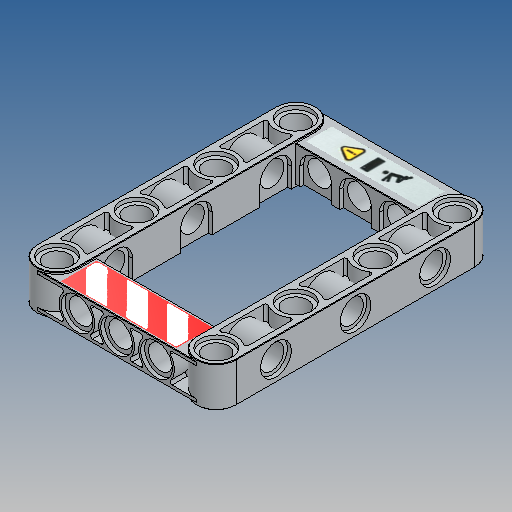
# Autodesk Inventor part: 64179-LtBluishGray
Saved by Autodesk Inventor 2025 (Build 290162010, 162A)
## iProperties
Created: 2012-03-21
Part Number: 64179-LtBluishGray
Document SubType Name: Modeling
Designer: D. Kohfeld
Density: 1.06 g/cm^3
Material: ABS Plastic
Mass: 5.69641 g
Surface Area: 80.0064 cm^2
Volume: 5.37397 cm^3
Appearance: LtBluishGray
Author: D. Kohfeld
Autodesk Inventor part; units mm, degrees
ref_plane "XZ Plane" through (0, 0, 0) normal (0, 1, 0) x (-1, 0, 0)
ref_plane "XY Plane" through (0, 0, 0) normal (0, 0, 1) x (1, 0, 0)
sketch "Sketch1" plane through (0, 0, 0) normal (0, 0, 1) x (1, 0, 0)
  line L0 (4, -24) -> (4, 24)
  line L1 (-4, 24) -> (-4, -24)
  arc A0 (4, 24) -> (-4, 24) centre (0, 24) ccw
  arc A1 (-4, -24) -> (4, -24) centre (0, -24) ccw
  circle A2 centre (0, 24) radius 3.2
  circle A3 centre (0, 24) radius 2.4
  line L2 (2.8284, 21.1716) -> (2.8284, 10.8284)
  line L3 (-2.8284, 21.1716) -> (-2.8284, 10.8284)
  arc A4 (-2.8284, 21.1716) -> (2.8284, 21.1716) centre (0, 24) ccw
  arc A5 (2.8284, 10.8284) -> (-2.8284, 10.8284) centre (0, 8) ccw
  circle A6 centre (0, 8) radius 3.2
  circle A7 centre (0, 8) radius 2.4
  line L4 (2.8284, 5.1716) -> (2.8284, -5.1716)
  line L5 (-2.8284, 5.1716) -> (-2.8284, -5.1716)
  arc A8 (-2.8284, 5.1716) -> (2.8284, 5.1716) centre (0, 8) ccw
  arc A9 (2.8284, -5.1716) -> (-2.8284, -5.1716) centre (0, -8) ccw
  circle A10 centre (0, -8) radius 3.2
  circle A11 centre (0, -8) radius 2.4
  line L6 (2.8284, -10.8284) -> (2.8284, -21.1716)
  line L7 (-2.8284, -10.8284) -> (-2.8284, -21.1716)
  arc A12 (-2.8284, -10.8284) -> (2.8284, -10.8284) centre (0, -8) ccw
  arc A13 (2.8284, -21.1716) -> (-2.8284, -21.1716) centre (0, -24) ccw
  circle A14 centre (0, -24) radius 3.2
  circle A15 centre (0, -24) radius 2.4
  line L8 (0, 24) -> (-2.8284, 21.1716) construction
  point P0 (0, 0)
  point P1 (-4, 0)
  dimension "d48" = 48
  dimension "d49" = 6.4
  dimension "d50" = 4.8
  dimension "d51" = 16
  dimension "d64" = 16
  dimension "d116" = 45
  dimension "d117" = 56
  dimension "d118" = 8
  constraints: 18 end point, 16 centre point, 16 point on circle, 9 coincident, 4 equal radius, 4 tangent, 3 horizontal alignment, 3 vertical, 2 vertical alignment, 1 midpoint, 1 parallel, 28 other
  measures "d48" distance of A1.centre A0.centre
  measures "d49" diameter of A2
  measures "d50" diameter of A3
  measures "d51" distance of A0.centre A5.centre
  measures "d64" distance of L3.start L5.start
  measures "d116" angle of L8 L1
  measures "d118" diameter of A0
extrude "Extrusion1" add sketch "Sketch1" along normal mid plane 8 contours A1 L1 A0 L0 | A2 | L2 A5 L3 A4 | A6 | L4 A9 L5 A8 | A10 | L6 A13 L7 A12 | A14
sketch "Sketch6" plane through (0, 0, 4) normal (0, 0, 1) x (1, 0, 0)
  circle A0 centre (0, 24) radius 2.4 projected
  circle A1 centre (0, 24) radius 3.2 projected
  line L0 (2.8284, 21.1716) -> (2.8284, 10.8284) projected
  arc A2 (-2.8284, 21.1716) -> (2.8284, 21.1716) centre (0, 24) ccw projected
  arc A3 (2.8284, 10.8284) -> (-2.8284, 10.8284) centre (0, 8) ccw projected
  line L1 (-2.8284, 21.1716) -> (-2.8284, 10.8284) projected
  circle A4 centre (0, 8) radius 3.2 projected
  circle A5 centre (0, 24) radius 3.1 projected
  circle A6 centre (0, 8) radius 3.1 projected
  line L2 (4, 24) -> (4, -24) projected
  line L3 (4, -24) -> (4, 24) projected
  arc A7 (-2.8284, 5.1716) -> (2.8284, 5.1716) centre (0, 8) ccw projected
  line L4 (2.8284, 5.1716) -> (2.8284, -5.1716) projected
  arc A8 (2.8284, -5.1716) -> (-2.8284, -5.1716) centre (0, -8) ccw projected
  line L5 (-2.8284, 5.1716) -> (-2.8284, -5.1716) projected
  circle A9 centre (0, -8) radius 3.2 projected
  line L6 (2.8284, -10.8284) -> (2.8284, -21.1716) projected
  arc A10 (-2.8284, -10.8284) -> (2.8284, -10.8284) centre (0, -8) ccw projected
  line L7 (-2.8284, -10.8284) -> (-2.8284, -21.1716) projected
  arc A11 (2.8284, -21.1716) -> (-2.8284, -21.1716) centre (0, -24) ccw projected
  circle A12 centre (0, -24) radius 3.2 projected
extrude "Extrusion7" cut sketch "Sketch6" against normal blind 0.8 contours A0 | A1 | A4 | A5 | A6 | A9 | A12
extrude "Extrusion8" cut sketch "Sketch6" against normal blind 3.1 contours L0 A3 L1 A2 | A7 L4 A8 L5 | L6 A11 L7 A10
sketch "Sketch15" plane through (0, 0, -4) normal (0, 0, -1) x (-1, 0, 0)
  circle A0 centre (0, -8) radius 2.4 projected
  circle A1 centre (0, 8) radius 2.4 projected
  arc A2 (4, 24) -> (-4, 24) centre (0, 24) ccw projected
  line L0 (-4, -24) -> (-4, 24) projected
  arc A3 (-4, -24) -> (4, -24) centre (0, -24) ccw projected
  line L1 (4, 24) -> (4, -24) projected
  line L2 (-2.8284, -5.1716) -> (-2.8284, 5.1716)
  arc A4 (2.4, -4.8) -> (-2.8284, -5.1716) centre (0, -8) ccw
  arc A5 (-2.8284, 5.1716) -> (2.4, 4.8) centre (0, 8) ccw
  line L3 (2.4, 4.8) -> (2.4, -4.8)
  line L4 (0, -8) -> (-2.8284, -5.1716) construction
  line L5 (-2.8284, -21.1716) -> (-2.8284, -10.8284)
  line L6 (2.4, -20.8) -> (2.4, -11.2)
  arc A6 (2.4, -20.8) -> (-2.8284, -21.1716) centre (0, -24) ccw
  arc A7 (-2.8284, -10.8284) -> (2.4, -11.2) centre (0, -8) ccw
  line L7 (-2.8284, 10.8284) -> (-2.8284, 21.1716)
  line L8 (2.4, 11.2) -> (2.4, 20.8)
  arc A8 (2.4, 11.2) -> (-2.8284, 10.8284) centre (0, 8) ccw
  arc A9 (-2.8284, 21.1716) -> (2.4, 20.8) centre (0, 24) ccw
  point P0 (0, 0)
  dimension "d109" = 45
  dimension "d111" = 1.6
  constraints: 14 end point, 12 point on circle, 6 centre point, 6 coincident, 6 equal radius, 6 parallel, 4 vertical alignment, 1 vertical
  measures "d109" angle of L0 L4
  measures "d111" distance between parallel lines of L1 L6
extrude "Extrusion19" cut sketch "Sketch15" against normal blind 3.1 contours L2 A5 L3 A4 | L5 A7 L6 A6 | L7 A9 L8 A8
mirror "Mirror5" about plane through (0, 0, 0) normal (0, 0, 1) of "Extrusion7"
sketch "Sketch7" plane through (0, 0, 0) normal (1, 0, 0) x (0, 1, 0)
  circle A0 centre (-16, 0) radius 3.6
  circle A1 centre (-16, 0) radius 2.4
  circle A2 centre (0, 0) radius 3.6
  circle A3 centre (0, 0) radius 2.4
  circle A4 centre (16, 0) radius 3.6
  circle A5 centre (16, 0) radius 2.4
  line L0 (-16, 0) -> (0, 0) construction
  line L1 (0, 0) -> (16, 0) construction
  dimension "d69" = 7.2
  dimension "d70" = 4.8
  dimension "d114" = 16
  constraints: 6 centre point, 4 coincident, 4 end point, 4 equal radius, 2 collinear, 1 horizontal alignment
  measures "d69" diameter of A0
  measures "d70" diameter of A1
  measures "d114" distance of L0.start L0.end
extrude "Extrusion9" add sketch "Sketch7" against normal up to surface (8 mm away) from surface at 4
extrude "Extrusion10" cut sketch "Sketch7" along normal through all both and the other way through all contours A1 | A3 | A5
sketch "Sketch8" plane through (4, -24, 4) normal (1, 0, 0) x (0, 0, -1)
  circle A0 centre (4, 24) radius 2.4 projected
  circle A1 centre (4, 8) radius 2.4 projected
  circle A2 centre (4, 40) radius 2.4 projected
  circle A3 centre (4, 8) radius 3.1
  circle A4 centre (4, 24) radius 3.1
  circle A5 centre (4, 40) radius 3.1
  dimension "d75" = 6.2
  constraints: 3 centre point, 3 coincident, 2 equal radius
  measures "d75" diameter of A3
extrude "Extrusion11" cut sketch "Sketch8" against normal blind 0.8
sketch "Sketch14" plane through (-4, -24, 4) normal (-1, 0, 0) x (0, 0, 1)
  circle A0 centre (-4, 24) radius 2.4 projected
  circle A1 centre (-4, 8) radius 2.4 projected
  circle A2 centre (-4, 40) radius 2.4 projected
  line L0 (-8, 48) -> (-8, 0) projected
  line L1 (-8, 0) -> (0, 0) projected
  line L2 (-8, 43.2) -> (-4, 43.2)
  arc A3 (-4, 36.8) -> (-4, 43.2) centre (-4, 40) ccw
  line L3 (-4, 36.8) -> (-8, 36.8)
  line L4 (-8, 27.2) -> (-4, 27.2)
  arc A4 (-4, 20.8) -> (-4, 27.2) centre (-4, 24) ccw
  line L5 (-4, 20.8) -> (-8, 20.8)
  line L6 (-8, 11.2) -> (-4, 11.2)
  arc A5 (-4, 4.8) -> (-4, 11.2) centre (-4, 8) ccw
  line L7 (-4, 4.8) -> (-8, 4.8)
  dimension "d106" = 6.4
  constraints: 12 end point, 6 point on circle, 6 point on line, 6 tangent, 3 centre point, 3 concentric, 3 parallel, 3 perpendicular, 2 equal radius
  measures "d106" diameter of A3
extrude "Extrusion18" cut sketch "Sketch14" against normal blind 0.8
fillet "Fillet2" radius 0.4 24 edges at (-2.8284, 21.1716, 2.45) (-2.8284, 10.8284, 2.45) (2.8284, 10.8284, 2.45) (2.8284, 21.1716, 2.45) (-2.8284, -21.1716, 2.45) (-2.8284, -10.8284, 2.45) (2.8284, -10.8284, 2.45) (2.8284, -21.1716, 2.45) (2.8284, -5.1716, 2.45) (-2.8284, -5.1716, 2.45) (-2.8284, 5.1716, 2.45) (2.8284, 5.1716, 2.45) (-2.4, 20.8, -2.45) (2.8284, 21.1716, -2.45) (2.8284, 10.8284, -2.45) (-2.4, 11.2, -2.45) (-2.4, 4.8, -2.45) (2.8284, 5.1716, -2.45) (-2.4, -4.8, -2.45) (2.8284, -5.1716, -2.45) (-2.4, -11.2, -2.45) (2.8284, -10.8284, -2.45) (2.8284, -21.1716, -2.45) (-2.4, -20.8, -2.45)
fillet "Fillet2" radius 0.1 11 edges at (-4, 0, 4) (0, 28, 4) (4, 0, 4) (0, -28, 4) (0, 28, -4) (-4, 8, -4) (-4, -8, -4) (-4, -21.6, -4) (-4, 21.6, -4) (0, -28, -4) (4, 0, -4)
ref_plane "Work Plane1" through (-16, 0, 0) normal (1, 0, 0) x (0, 1, 0)
sketch "Sketch11" plane through (-16, 0, 0) normal (1, 0, 0) x (0, 1, 0)
  line L0 (-28, -3.9) -> (-28, 3.9) construction
  line L1 (-28, -3.6) -> (-20, -3.6)
  line L2 (-20, -3.6) -> (-20, 3.6)
  line L3 (-20, 3.6) -> (-28, 3.6)
  line L4 (-28, 3.6) -> (-28, 2.9)
  line L5 (-28, 2.9) -> (-24.9, 2.9)
  line L6 (-24.9, 2.9) -> (-24.9, -2.9)
  line L7 (-24.9, -2.9) -> (-28, -2.9)
  line L8 (-28, -2.9) -> (-28, -3.6)
  point P0 (0, 0)
  point P1 (-20, 0)
  point P2 (-28, 0)
  dimension "d86" = 8
  dimension "d87" = 3.1
  dimension "d88" = 5.8
  dimension "d89" = 7.2
  constraints: 16 end point, 6 perpendicular, 4 point on line, 2 collinear, 2 midpoint, 1 horizontal alignment
  measures "d86" distance between parallel lines of L2 L0
  measures "d87" distance between parallel lines of L0 L6
  measures "d88" distance between parallel lines of L7 L5
  measures "d89" distance between parallel lines of L1 L3
extrude "Extrusion13" add sketch "Sketch11" along normal up to next
sketch "Sketch12" plane through (-16, -28, 2.9) normal (0, -1, 0) x (1, 0, 0)
  line L0 (0, 0.7) -> (16, 0.7) projected
  line L1 (0, 0.7) -> (0, 0) projected
  line L2 (16, -6.5) -> (16, -5.8) projected
  line L3 (0, -5.8) -> (16, -5.8) projected
  line L4 (0, -5.8) -> (0, -6.5) projected
  line L5 (0, -6.5) -> (16, -6.5) projected
  circle A0 centre (8, -2.9) radius 3.6
  circle A1 centre (8, -2.9) radius 2.4
  circle A2 centre (8, -2.9) radius 3.2
  arc A3 (0, -6.5) -> (0, 0.7) centre (0, -2.9) ccw
  arc A4 (0, -6.1) -> (0, 0.3) centre (0, -2.9) ccw
  circle A5 centre (0, -2.9) radius 2.4
  line L6 (0, -2.9) -> (8, -2.9) construction
  line L7 (8, -2.9) -> (16, -2.9) construction
  line L8 (0, -6.5) -> (0, 0.7)
  dimension "d92" = 4.8
  dimension "d93" = 6.4
  constraints: 6 centre point, 6 end point, 4 coincident, 4 point on circle, 4 tangent, 3 collinear, 2 equal radius, 2 point on line, 1 horizontal alignment, 1 parallel
  measures "d92" diameter of A5
  measures "d93" diameter of A4
extrude "Extrusion14" add sketch "Sketch12" against normal up to surface (3.1 mm away) contours A3 L3 A4 L1 | A0 L3 A2 | A4 L3 L8 A5 L1 | A3 L4 A4 L3 | L3 A2 A0 | A4 L4 L3 | A2 L3 | L3 A2 | A5 L8 picked at (0.4988, -2.2745)
extrude "Extrusion15" cut sketch "Sketch12" against normal through all contours L8 A5 | A5 L8 | A1
extrude "Extrusion16" cut sketch "Sketch12" against normal blind 0.8 contours A4 L3 L8 A5 L1 | A4 L4 L3 | A2 L3 | L3 A2 | A5 L8 picked at (0.4988, -2.2745)
sketch "Sketch13" plane through (-16, -20, 3.6) normal (0, 1, 0) x (1, 0, 0)
  arc A0 (0, 1.2) -> (0, 6) centre (0, 3.6) ccw projected
  line L0 (0, 1.2) -> (0, 0) projected
  line L1 (0, 7.2) -> (12, 7.2) projected
  line L2 (0, 7.2) -> (0, 6) projected
  circle A1 centre (8, 3.6) radius 2.4 projected
  line L3 (3.2, 7.2) -> (3.2, 3.6)
  arc A2 (0, 0.4) -> (3.2, 3.6) centre (0, 3.6) ccw
  arc A3 (4.8, 3.6) -> (11.2, 3.6) centre (8, 3.6) ccw
  line L4 (4.8, 3.6) -> (4.8, 7.2)
  line L5 (11.2, 3.6) -> (11.2, 7.2)
  point P0 (16, 3.6)
  dimension "d100" = 6.4
  constraints: 6 end point, 4 point on circle, 4 point on line, 3 tangent, 2 centre point, 2 coincident, 2 perpendicular, 1 equal radius, 1 parallel
  measures "d100" diameter of A3
extrude "Extrusion17" cut sketch "Sketch13" against normal blind 0.8
fillet "Fillet3" radius 0.1 7 edges at (-4, -28, 3.6) (-12, -28, 3.6) (-10, -20, 3.6) (-12, -28, -3.6) (-4, -28, -3.6) (-4.4, -20, -3.6) (-12, -20, -3.6)
fillet "Fillet3" radius 0.4 6 edges at (-5.8669, -26.45, -2.9) (-5.8669, -26.45, 2.9) (-10.1331, -26.45, 2.9) (-10.1331, -26.45, -2.9) (-13.8669, -26.45, -2.9) (-13.8669, -26.45, 2.9)
mirror "Mirror4" about plane through (0, 0, 0) normal (0, 1, 0) of "Extrusion13", "Extrusion14", "Extrusion16", "Extrusion17", "Extrusion15", "Fillet3"
mirror "Mirror3" about plane through (-16, 0, 0) normal (1, 0, 0) of "Extrusion7", "Extrusion1", "Extrusion11", "Extrusion10", "Extrusion9", "Extrusion8", "Fillet2", "Extrusion13", "Extrusion14", "Extrusion16", "Extrusion17", "Extrusion15", "Mirror4", "Fillet3", "Extrusion19", "Extrusion18", "Mirror5"
sketch "Skizze16" plane through (-4, -24, 3.6) normal (0, 0, 1) x (1, 0, 0)
  line L0 (-23.3393, 50.6) -> (-0.6607, 50.6) construction
  line L1 (-0.6607, 50.6) -> (-0.6607, 45.4) construction
  line L2 (-0.6607, 45.4) -> (-23.3393, 45.4) construction
  line L3 (-23.3393, 45.4) -> (-23.3393, 50.6) construction
  line L4 (-28, -4) -> (4, -4) projected
  line L5 (4, 52) -> (-28, 52) projected
  line L6 (-24, 44) -> (0, 44) projected
  line L7 (-27.1112, 51.9) -> (3.1112, 51.9) projected
  point P0 (4, 24)
  point P1 (-12, 50.6)
  point P2 (-14.8102, 48.9)
  point P3 (-12, 51.9)
  dimension "d146" = 1.4
  dimension "d147" = 1.4
  constraints: 2 midpoint, 1 vertical alignment, 2 other
  measures "d146" distance between parallel lines of L5 L0
  measures "d147" distance between parallel lines of L2 L6
decal "Aufkleber1"
sketch "Skizze17" plane through (-4, 20.1, 3.6) normal (0, 0, 1) x (1, 0, 0)
  line L0 (-23.6033, -40.5) -> (-0.3967, -40.5) construction
  line L1 (-0.3967, -40.5) -> (-0.3967, -47.7) construction
  line L2 (-0.3967, -47.7) -> (-23.6033, -47.7) construction
  line L3 (-23.6033, -47.7) -> (-23.6033, -40.5) construction
  line L4 (0, -40.1) -> (-24, -40.1) projected
  line L5 (-28, -48.1) -> (4, -48.1) projected
  point P0 (4, -20.1)
  point P1 (-12, -47.7)
  point P2 (-12, -40.1)
  dimension "d154" = 0.4
  dimension "d157" = 0.4
  constraints: 2 midpoint, 1 vertical alignment, 2 other
  measures "d154" distance between parallel lines of L4 L0
  measures "d157" distance between parallel lines of L2 L5
decal "Aufkleber2"
equation "\"lf\" = 0.1"
equation "\"tf\" = 0.4"
body "Solid1"
